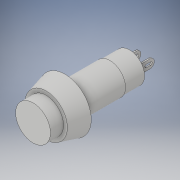
# Autodesk Inventor part: przycisk
Saved by Autodesk Inventor 2019 (Build 230136000, 136)
## iProperties
Created: 2019-09-16
Part Number: przycisk
Material: Ogólny
Document SubType Name: Modeling
Designer: mikol
Density: 1 g/cm^3
Appearance: Domyślna
Author: mikol
Autodesk Inventor part; units mm, degrees
ref_plane "YZ Plane" through (0, 0, 0) normal (1, 0, 0) x (0, 1, 0)
ref_plane "XZ Plane" through (0, 0, 0) normal (0, 1, 0) x (-1, 0, 0)
ref_plane "XY Plane" through (0, 0, 0) normal (0, 0, 1) x (1, 0, 0)
sketch "Sketch1" plane through (0, 0, 0) normal (0, 0, 1) x (1, 0, 0)
  circle A0 centre (0, 0) radius 5.175
  dimension "d0" = 10.35
  constraints: 1 centre point, 1 coincident
  measures "d0" diameter of A0
extrude "Extrusion1" add sketch "Sketch1" along normal blind 6.75
sketch "Sketch2" plane through (0, 0, 6.75) normal (0, 0, 1) x (1, 0, 0)
  circle A0 centre (0, 0) radius 5.375
  dimension "d3" = 10.75
  constraints: 1 centre point, 1 coincident
  measures "d3" diameter of A0
extrude "Extrusion2" add sketch "Sketch2" along normal blind 15.5
sketch "Sketch3" plane through (0, 0, 22.25) normal (0, 0, 1) x (1, 0, 0)
  circle A0 centre (0, 0) radius 9.05
  dimension "d6" = 18.1
  constraints: 1 centre point, 1 coincident
  measures "d6" diameter of A0
extrude "Extrusion3" add sketch "Sketch3" along normal blind 6.5
chamfer "Chamfer1" distance 6.5 angle 15 1 edges at (-9.05, 0, 28.75) measured on face at (8.9328, -1.4517, 26.5833)
sketch "Sketch4" plane through (0, 0, 0) normal (0, 0, -1) x (-1, 0, 0)
  circle A0 centre (0, 0) radius 5.175 projected
  line L0 (2.55, 1.5) -> (2.05, 1.5)
  line L1 (2.05, 1.5) -> (2.05, -1.5)
  line L2 (2.05, -1.5) -> (2.55, -1.5)
  line L3 (2.55, -1.5) -> (2.55, 1.5)
  line L4 (-2.05, 1.5) -> (-2.55, 1.5)
  line L5 (-2.55, 1.5) -> (-2.55, -1.5)
  line L6 (-2.55, -1.5) -> (-2.05, -1.5)
  line L7 (-2.05, -1.5) -> (-2.05, 1.5)
  dimension "d12" = 0.5
  dimension "d13" = 3
  dimension "d14" = 0.5
  dimension "d15" = 3
  dimension "d16" = 5.1
  dimension "d17" = 2.625
  dimension "d18" = 2.625
  dimension "d19" = 3.675
  dimension "d20" = 3.675
  constraints: 16 end point, 4 parallel, 2 horizontal, 2 perpendicular, 1 point on line
  measures "d12" distance of L2.end L1.end
  measures "d13" distance of L1.end L0.end
  measures "d14" distance of L6.end L5.end
  measures "d15" distance of L5.end L4.end
  measures "d16" distance between parallel lines of L5 L3
  measures "d17" distance edge to line of A0 L3
  measures "d18" distance edge to line of A0 L5
  measures "d19" distance edge to line of A0 L0
  measures "d20" distance edge to line of A0 L2
extrude "Extrusion4" add sketch "Sketch4" along normal blind 6 contours L3 L2 L1 L0 | L7 L6 L5 L4
fillet "Fillet1" radius 1.5 4 edges at (-2.3, 1.5, -6) (-2.3, -1.5, -6) (2.3, 1.5, -6) (2.3, -1.5, -6)
sketch "Sketch5" plane through (-2.55, -1.5, 0) normal (-1, 0, 0) x (0, 0, 1)
  line L0 (-4.7053, 1.5) -> (-3.2606, 1.5) construction
  line L1 (-4.7053, 0.9641) -> (-3.2606, 0.9641)
  line L2 (-3.2606, 2.0359) -> (-4.7053, 2.0359)
  arc A0 (-4.7053, 2.0359) -> (-4.7053, 0.9641) centre (-4.7053, 1.5) ccw
  arc A1 (-3.2606, 0.9641) -> (-3.2606, 2.0359) centre (-3.2606, 1.5) ccw
  line L3 (0, 0) -> (-4.5, 0) projected
  line L4 (0, 3) -> (-4.5, 3) projected
  point P0 (0, 1.5)
  point P1 (-3.983, 1.5)
  dimension "d24" = 1.5
  dimension "d25" = 1.5
  constraints: 8 end point, 4 point on circle, 4 tangent, 2 centre point, 1 horizontal, 1 midpoint, 1 parallel
  measures "d24" distance from line of L3 L0.start
  measures "d25" distance from line of L4 L0.start
extrude "Extrusion5" cut sketch "Sketch5" against normal through all
sketch "Sketch6" plane through (0, 0, 28.75) normal (0, 0, 1) x (1, 0, 0)
  circle A0 centre (0, 0) radius 6
  dimension "d28" = 12
  constraints: 1 centre point, 1 coincident
  measures "d28" diameter of A0
extrude "Extrusion6" add sketch "Sketch6" along normal blind 4.5
equation "\"d17\" = d18"
equation "\"d19\" = d20"
equation "\"d24\" = d25"
body "Solid1"
